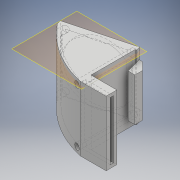
# Autodesk Inventor part: CarroXY - Ventilador
Saved by Autodesk Inventor 2017 (Build 210142000, 142)
## iProperties
Created: 2020-09-26
Part Number: CarroXY - Ventilador
Material: Generic
Document SubType Name: Modeling
Designer: ale
Density: 1 g/cm^3
Appearance: Default
Author: ale
Autodesk Inventor part; units mm, degrees
ref_plane "YZ Plane" through (0, 0, 0) normal (1, 0, 0) x (0, 1, 0)
ref_plane "XZ Plane" through (0, 0, 0) normal (0, 1, 0) x (-1, 0, 0)
ref_plane "XY Plane" through (0, 0, 0) normal (0, 0, 1) x (1, 0, 0)
sketch "Sketch1" plane through (0, 0, 0) normal (0, 0, 1) x (1, 0, 0)
  line L0 (-7, 0) -> (-48, 0)
  line L1 (0, -7) -> (-7, 0)
  line L2 (-64.3371, -29.6543) -> (-6.3816, -14.1252)
  line L3 (-6.3816, -14.1252) -> (-9.2286, -3.5)
  line L4 (-9.2286, -3.5) -> (-67.1841, -19.0291)
  line L5 (-67.1841, -19.0291) -> (-64.3371, -29.6543)
  line L6 (-3.5, -3.5) -> (4.0544, 4.0544)
  line L7 (0, -14.1252) -> (0, -7)
  line L8 (-7, 0) -> (-17, 0)
  line L9 (-17, 0) -> (-17, -5.5823)
  line L10 (-17, -5.5823) -> (-9.2286, -3.5)
  line L11 (-9.2286, -3.5) -> (-6.3816, -14.1252)
  line L12 (-6.3816, -14.1252) -> (0, -14.1252)
  line L13 (0, -14.1252) -> (0, -7)
  line L14 (0, -7) -> (-7, 0)
  line L15 (-7, 0) -> (-17, 0)
  point P0 (0, 0)
  dimension "d1" = 48
  dimension "d2" = 7
  dimension "d3" = 7
  dimension "d4" = 60
  dimension "d5" = 11
  dimension "d7" = 10
  constraints: 32 end point, 5 perpendicular, 3 collinear, 3 point on line, 2 parallel, 1 horizontal, 1 midpoint
  measures "d1" distance of point (0, 0) L0.end
  measures "d2" distance of L1.start point (0, 0)
  measures "d3" distance of L0.start point (0, 0)
  measures "d4" distance of L4.end L3.end
  measures "d5" distance of L3.end L2.end
  measures "d7" distance of L0.start L8.end
extrude "Extrusion1" add sketch "Sketch1" against normal blind 40 contours L1 L7 L12 L3 L4 L9 L0
sketch "Sketch2" plane through (-17, -5.5823, -40) normal (0.258819, -0.9659258, 0) x (0.9659258, 0.258819, 0)
  line L0 (8.0456, 40) -> (8.0456, 0) projected
  line L1 (8.0456, 20) -> (-21.9544, 20)
  line L2 (-51.9544, 50) -> (8.0456, 50)
  line L3 (8.0456, 50) -> (8.0456, -10)
  line L4 (8.0456, -10) -> (-51.9544, -10)
  line L5 (-51.9544, -10) -> (-51.9544, 50)
  line L6 (-51.9544, 50) -> (8.0456, -10) construction
  line L7 (8.0456, 50) -> (-51.9544, -10) construction
  circle A0 centre (-21.9544, 20) radius 28
  point P0 (17.8656, 40)
  dimension "d10" = 30
  dimension "d11" = 60
  dimension "d12" = 60
  dimension "d13" = 56
  constraints: 14 end point, 3 midpoint, 2 horizontal, 2 parallel, 1 centre point, 1 coincident, 1 perpendicular
  measures "d10" distance of L1.start L1.end
  measures "d11" distance of L3.end L4.end
  measures "d12" distance of L2.end L3.end
  measures "d13" diameter of A0
extrude "Extrusion2" add sketch "Sketch2" against normal blind 4
sketch "Sketch3" plane through (-7, 0, 0) normal (0, 1, 0) x (1, 0, 0)
  line L0 (7, 0) -> (0, 0) projected
  line L1 (0, 0) -> (-10, 0)
  line L2 (-10, 0) -> (-10, 40)
  line L3 (-10, 40) -> (0, 40)
  line L4 (0, 40) -> (0, 0)
  constraints: 8 end point, 2 parallel, 1 horizontal, 1 perpendicular
extrude "Extrusion3" cut sketch "Sketch3" along normal blind 4
sketch "Sketch4" plane through (-67.1841, -19.0291, 10) normal (0, 0, 1) x (0.9659258, 0.258819, 0)
  line L0 (53.0262, 4) -> (51.9544, 0) projected
  line L1 (60, 3.9999) -> (45.7649, -49.1261)
  line L2 (53.0262, 4) -> (108.0263, 4) construction
  line L3 (60, 0) -> (0, 0) projected
  line L4 (0, 0) -> (60, 0) projected
  arc A0 (0, 0) -> (45.7649, -49.1261) centre (92.7213, 40.4975) ccw
  line L5 (0, 0) -> (0, 4) projected
  line L6 (0, 0) -> (58.9282, 0)
  line L7 (58.9282, 0) -> (45.7649, -49.1261)
  point P0 (60, 4)
  dimension "d22" = 53.62
  dimension "d23" = 105
  constraints: 8 end point, 2 point on circle, 2 point on line, 1 centre point, 1 collinear, 1 equal length, 1 horizontal, 1 parallel
  measures "d22" distance of L0.start L1.end
  measures "d23" angle of L1 L2
extrude "Extrusion4" add sketch "Sketch4" against normal blind 60
ref_plane "Work Plane1" through (-10.2638, -54.6364, 7) normal (0, 0, 1) x (1, 0, 0)
sketch "Sketch5" plane through (-10.2638, -54.6364, 7) normal (0, 0, 1) x (1, 0, 0)
  line L0 (-57.9556, 39.471) -> (0, 55.0001)
  line L1 (0, 0) -> (0, 50.859) projected
  line L2 (0, 55.0001) -> (0, 0)
  line L3 (-56.9203, 35.6073) -> (-57.9556, 39.471) projected
  line L4 (-57.9556, 39.471) -> (-56.9203, 35.6073)
  arc A0 (-56.9203, 35.6073) -> (0, 0) centre (22.1601, 98.723) ccw
  line L5 (-3, 3.822) -> (-3, 51.0905)
  line L6 (-3, 51.0905) -> (-54.2813, 37.3497)
  line L7 (-54.2813, 37.3497) -> (-54.1859, 36.9937)
  arc A1 (-54.1859, 36.9937) -> (-3, 3.822) centre (22.1601, 98.723) ccw
  point P0 (10.2638, 54.6364)
  dimension "d1" = 48
  dimension "d2" = 7
  dimension "d3" = 7
  dimension "d4" = 60
  dimension "d5" = 11
  dimension "d7" = 10
  dimension "d27" = 3
  constraints: 12 end point, 4 point on circle, 2 centre point, 2 collinear, 3 other
  measures "d27" radial gap between concentric circles of A0 A1
extrude "Extrusion5" cut sketch "Sketch5" against normal blind 54 contours A1 L7 L6 L5
sketch "Sketch7" plane through (-10.2638, -54.6364, 10) normal (1, 0, 0) x (0, 0, -1)
  line L0 (0, 0) -> (0, 50.859) projected
  line L1 (60, 0) -> (60, 35.6073) projected
  line L2 (0, 0) -> (60, 0)
  line L3 (60, 0) -> (60, 10)
  line L4 (60, 10) -> (0, 10)
  line L5 (0, 10) -> (0, 0)
  point P0 (10, 54.6364)
  dimension "d38" = 10
  constraints: 8 end point, 2 parallel, 1 horizontal, 1 perpendicular, 1 point on line
  measures "d38" distance of L3.end L2.end
extrude "Extrusion7" add sketch "Sketch7" along normal blind 24
sketch "Sketch8" plane through (13.7362, -54.6364, 10) normal (1, 0, 0) x (0, 0, -1)
  line L0 (3, 36.9937) -> (3, 3.822) projected
  line L1 (3, 3.822) -> (57, 3.822)
  line L2 (57, 3.822) -> (57, 6.822)
  line L3 (57, 6.822) -> (3, 6.822)
  line L4 (3, 6.822) -> (3, 3.822)
  point P0 (10, 54.6364)
  dimension "d41" = 54
  dimension "d42" = 3
  constraints: 8 end point, 2 parallel, 1 horizontal, 1 perpendicular
  measures "d41" distance of L3.end L2.end
  measures "d42" distance of L2.end L1.end
extrude "Extrusion8" cut sketch "Sketch8" against normal up to next
sketch "Sketch9" plane through (-7, 0, 0) normal (0, 1, 0) x (1, 0, 0)
  line L0 (-57.2416, -5) -> (-7.2416, -5)
  line L1 (-7.2416, -5) -> (-7.2416, 45)
  line L2 (-7.2416, 45) -> (-57.2416, 45)
  line L3 (-57.2416, 45) -> (-57.2416, -5)
  arc A0 (-10.0192, 37.0343) -> (-24.8254, 47) centre (-32.2416, 20) ccw
  line L4 (-57.2416, -5) -> (-7.2416, 45) construction
  line L5 (-7.2416, -5) -> (-57.2416, 45) construction
  ellipse E0 centre (-32.2416, 20) end of major axis (-32.2416, 48) minor radius 27.0459 (-10, 35.9309) -> (-10, 4.0691) ccw projected
  point P0 (7.5784, 0)
  dimension "d45" = 50
  dimension "d46" = 50
  constraints: 12 end point, 4 coincident, 2 midpoint, 2 parallel, 2 point on circle, 1 centre point, 1 horizontal, 1 perpendicular, 1 other
  measures "d45" distance of L2.end L1.end
  measures "d46" distance of L1.end L0.end
hole "Hole1" at (-64.2416, 0, 5) at (-14.2416, 0, -45) at (-14.2416, 0, 5) at (-64.2416, 0, -45) direction (0, -1, 0) diameter 5.5 end through all
equation "\"d3\" = d2"
body "Solid1"
